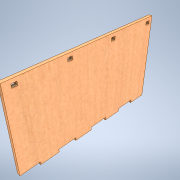
# Autodesk Inventor part: DoosjeRechterkant
Saved by Autodesk Inventor 2021 (Build 250183000, 183)
## iProperties
Created: 2021-03-11
Part Number: DoosjeRechterkant
Material: Wood (Cherry)
Document SubType Name: Modeling
Designer: ZiweZhang
Density: 0.63 g/cm^3
Appearance: Cherry - Natural Low Gloss
Author: ZiweZhang
Autodesk Inventor part; units mm, degrees
ref_plane "YZ Plane" through (0, 0, 0) normal (1, 0, 0) x (0, 1, 0)
ref_plane "XZ Plane" through (0, 0, 0) normal (0, 1, 0) x (-1, 0, 0)
ref_plane "XY Plane" through (0, 0, 0) normal (0, 0, 1) x (1, 0, 0)
sketch "Sketch1" plane through (0, 0, 0) normal (1, 0, 0) x (0, 1, 0)
  line L0 (0, 0) -> (77, 0)
  line L1 (77, 0) -> (77, -140)
  line L2 (77, -140) -> (0, -140)
  line L3 (0, 0) -> (-3, 0)
  line L4 (-3, 0) -> (-3, -140)
  line L5 (-3, -140) -> (0, -140)
  dimension "d1" = 140
  constraints: 12 end point, 3 perpendicular, 2 horizontal, 1 parallel
  measures "d1" distance of L0.end L1.end
extrude "Extrusion1" add sketch "Sketch1" along normal blind 3
sketch "Sketch5" plane through (3, 0, 0) normal (1, 0, 0) x (0, 0, -1)
  line L0 (6, 73.9) -> (6, 70.9)
  line L1 (6, 70.9) -> (10, 70.9)
  line L2 (10, 70.9) -> (10, 73.9)
  line L3 (10, 73.9) -> (6, 73.9)
  line L4 (0, 77) -> (0, 0) projected
  line L5 (140, 77) -> (0, 77) projected
  line L6 (37.75, 73.9) -> (37.75, 70.9)
  line L7 (37.75, 70.9) -> (41.75, 70.9)
  line L8 (41.75, 70.9) -> (41.75, 73.9)
  line L9 (41.75, 73.9) -> (37.75, 73.9)
  line L10 (6, 35.9) -> (6, 32.9)
  line L11 (6, 32.9) -> (10, 32.9)
  line L12 (10, 32.9) -> (10, 35.9)
  line L13 (10, 35.9) -> (6, 35.9)
  line L14 (37.75, 35.9) -> (37.75, 32.9)
  line L15 (37.75, 32.9) -> (41.75, 32.9)
  line L16 (41.75, 32.9) -> (41.75, 35.9)
  line L17 (41.75, 35.9) -> (37.75, 35.9)
  line L18 (69.5, 73.9) -> (69.5, 70.9)
  line L19 (69.5, 70.9) -> (73.5, 70.9)
  line L20 (73.5, 70.9) -> (73.5, 73.9)
  line L21 (73.5, 73.9) -> (69.5, 73.9)
  line L22 (69.5, 35.9) -> (69.5, 32.9)
  line L23 (69.5, 32.9) -> (73.5, 32.9)
  line L24 (73.5, 32.9) -> (73.5, 35.9)
  line L25 (73.5, 35.9) -> (69.5, 35.9)
  line L26 (101.25, 73.9) -> (101.25, 70.9)
  line L27 (101.25, 70.9) -> (105.25, 70.9)
  line L28 (105.25, 70.9) -> (105.25, 73.9)
  line L29 (105.25, 73.9) -> (101.25, 73.9)
  line L30 (101.25, 35.9) -> (101.25, 32.9)
  line L31 (101.25, 32.9) -> (105.25, 32.9)
  line L32 (105.25, 32.9) -> (105.25, 35.9)
  line L33 (105.25, 35.9) -> (101.25, 35.9)
  line L34 (133, 73.9) -> (133, 70.9)
  line L35 (133, 70.9) -> (137, 70.9)
  line L36 (137, 70.9) -> (137, 73.9)
  line L37 (137, 73.9) -> (133, 73.9)
  line L38 (133, 35.9) -> (133, 32.9)
  line L39 (133, 32.9) -> (137, 32.9)
  line L40 (137, 32.9) -> (137, 35.9)
  line L41 (137, 35.9) -> (133, 35.9)
  line L42 (10, 26.8) -> (10, 29.8)
  line L43 (10, 29.8) -> (6, 29.8)
  line L44 (6, 26.8) -> (10, 26.8)
  line L45 (6, 29.8) -> (6, 26.8)
  line L46 (69.5, 29.8) -> (69.5, 26.8)
  line L47 (69.5, 26.8) -> (73.5, 26.8)
  line L48 (73.5, 29.8) -> (69.5, 29.8)
  line L49 (73.5, 26.8) -> (73.5, 29.8)
  line L50 (41.75, 29.8) -> (37.75, 29.8)
  line L51 (37.75, 26.8) -> (41.75, 26.8)
  line L52 (41.75, 26.8) -> (41.75, 29.8)
  line L53 (37.75, 29.8) -> (37.75, 26.8)
  line L54 (133, 29.8) -> (133, 26.8)
  line L55 (137, 29.8) -> (133, 29.8)
  line L56 (133, 26.8) -> (137, 26.8)
  line L57 (137, 26.8) -> (137, 29.8)
  line L58 (101.25, 29.8) -> (101.25, 26.8)
  line L59 (101.25, 26.8) -> (105.25, 26.8)
  line L60 (105.25, 26.8) -> (105.25, 29.8)
  line L61 (105.25, 29.8) -> (101.25, 29.8)
  line L62 (140, -3) -> (140, 77) projected
  dimension "d67" = 3
  dimension "d68" = 4
  dimension "d93" = 3.1
  dimension "d97" = 6
  dimension "d100" = 31.75
  dimension "d103" = 38
  dimension "d108" = 6.1
  dimension "d113" = 3
  constraints: 120 end point, 3 collinear, 3 perpendicular, 3 vertical, 1 horizontal, 109 other
  measures "d67" distance of L0.start L0.end
  measures "d68" distance of L0.end L1.end
  measures "d93" distance between parallel lines of L5 L3
  measures "d97" distance between parallel lines of L4 L0
  measures "d100" distance of L0.start L6.start
  measures "d103" distance of L0.start L10.start
  measures "d108" distance of L11.end L42.start
  measures "d113" distance between parallel lines of L62 L36
extrude "Extrusion5" cut sketch "Sketch5" against normal blind 10
sketch "Sketch6" plane through (3, 0, 0) normal (1, 0, 0) x (0, 0, -1)
  line L0 (0, 0) -> (17.5, 0)
  line L1 (17.5, 0) -> (17.5, -3)
  line L2 (17.5, -3) -> (35, -3)
  line L3 (35, -3) -> (35, 0)
  line L4 (0, 0) -> (0, 10)
  line L5 (140, 0) -> (140, 9.94)
  line L6 (137, 9.94) -> (137, 19.94)
  line L7 (137, 19.94) -> (140, 19.94)
  line L8 (140, 30) -> (137, 30)
  line L9 (137, 30) -> (137, 40)
  line L10 (137, 40) -> (140, 40)
  line L11 (140, 40) -> (140, 50)
  line L12 (140, 50) -> (137, 50)
  line L13 (137, 50) -> (137, 60)
  line L14 (137, 60) -> (140, 60)
  line L15 (140, 60) -> (140, 70)
  line L16 (140, 70) -> (137, 70)
  line L17 (137, 70) -> (137, 77)
  line L18 (140, 9.94) -> (137, 9.94)
  line L19 (140, 19.94) -> (140, 30)
  line L20 (3, 77) -> (137, 77)
  line L21 (0, 77) -> (0, 0)
  line L22 (0, 0) -> (0, 77)
  line L23 (0, 77) -> (3, 77)
  line L24 (35, 0) -> (52.5, 0)
  line L25 (52.5, 0) -> (52.5, -3)
  line L26 (52.5, -3) -> (70, -3)
  line L27 (70, -3) -> (70, 0)
  line L28 (70, 0) -> (87.5, 0)
  line L29 (87.5, 0) -> (87.5, -3)
  line L30 (87.5, -3) -> (105, -3)
  line L31 (105, -3) -> (105, 0)
  line L32 (105, 0) -> (122.5, 0)
  line L33 (122.5, 0) -> (122.5, -3)
  line L34 (122.5, -3) -> (140, -3)
  line L35 (140, 30) -> (140, 19.94)
  line L36 (140, 9.94) -> (140, -3)
  line L37 (140, 40) -> (140, 50)
  line L38 (140, 60) -> (140, 70)
  line L39 (140, -3) -> (140, 9.94)
  line L40 (137, 9.94) -> (137, 19.94)
  line L41 (0, 0) -> (0, 77)
  line L42 (137, 77) -> (0, 77)
  line L43 (0, 77) -> (0, 10)
  point P0 (0, 70)
  constraints: 88 end point, 16 point on line
extrude "Extrusion6" cut sketch "Sketch6" against normal blind 3 keep common part
body "Solid1"
